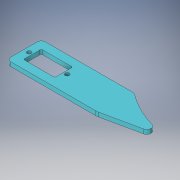
# Autodesk Inventor part: legRound
Saved by Autodesk Inventor 2019.1 (Build 231200000, 200)
## iProperties
Created: 2018-11-13
Part Number: legRound
Material: Generic
Document SubType Name: Modeling
Designer: kfortuna
Density: 1 g/cm^3
Appearance: Default
Author: kfortuna
Autodesk Inventor part; units mm, degrees
ref_plane "YZ Plane" through (0, 0, 0) normal (1, 0, 0) x (0, 1, 0)
ref_plane "XZ Plane" through (0, 0, 0) normal (0, 1, 0) x (-1, 0, 0)
ref_plane "XY Plane" through (0, 0, 0) normal (0, 0, 1) x (1, 0, 0)
sketch "Sketch1" plane through (0, 0, 0) normal (0, 1, 0) x (-1, 0, 0)
  line L0 (25.9896, 44.1273) -> (5.2671, 44.1273)
  line L1 (4.2671, 43.1273) -> (4.2671, 32.1273)
  line L2 (5.2671, 31.1273) -> (25.9896, 31.1273)
  line L3 (26.9896, 32.1273) -> (26.9896, 43.1273)
  line L4 (29.9896, 50.1273) -> (-31.3027, 50.1273)
  line L5 (-32.806, 25.1273) -> (29.9896, 25.1273)
  line L6 (32.9896, 28.1273) -> (32.9896, 47.1273)
  line L7 (-33.3897, 49.9071) -> (-60.206, 44.1846)
  arc A0 (-35.8175, 26.1359) -> (-60.3814, 38.2573) centre (-79.9609, -32.3705) ccw
  circle A1 centre (29.3148, 37.6273) radius 1.5
  circle A2 centre (1.7671, 37.6273) radius 1.5
  arc A3 (32.9896, 47.1273) -> (29.9896, 50.1273) centre (29.9896, 47.1273) ccw
  arc A4 (29.9896, 25.1273) -> (32.9896, 28.1273) centre (29.9896, 28.1273) ccw
  arc A5 (26.9896, 43.1273) -> (25.9896, 44.1273) centre (25.9896, 43.1273) ccw
  arc A6 (25.9896, 31.1273) -> (26.9896, 32.1273) centre (25.9896, 32.1273) ccw
  arc A7 (4.2671, 32.1273) -> (5.2671, 31.1273) centre (5.2671, 32.1273) ccw
  arc A8 (5.2671, 44.1273) -> (4.2671, 43.1273) centre (5.2671, 43.1273) ccw
  arc A9 (-35.8175, 26.1359) -> (-32.806, 25.1273) centre (-32.806, 30.1273) ccw
  arc A10 (-31.3027, 50.1273) -> (-33.3897, 49.9071) centre (-31.3027, 40.1273) ccw
  line L8 (-62.58, 41.2506) -> (-62.58, 41.1483)
  arc A11 (-60.206, 44.1846) -> (-62.58, 41.2506) centre (-59.58, 41.2506) ccw
  arc A12 (-62.58, 41.1483) -> (-60.3814, 38.2573) centre (-59.58, 41.1483) ccw
  point P0 (0, 0)
  point P1 (26.9896, 44.1273)
  point P2 (4.2671, 31.1273)
  point P3 (4.2671, 44.1273)
  point P4 (26.9896, 31.1273)
  point P5 (32.9896, 50.1273)
  point P6 (-34.5115, 25.1273)
  point P7 (-32.3578, 50.1273)
  point P8 (32.9896, 25.1273)
  point P9 (-62.58, 38.8302)
  dimension "d0" = 13
  dimension "d1" = 6
  dimension "d2" = 6
  dimension "d3" = 3
  dimension "d4" = 12.5
  dimension "d5" = 12.5
  dimension "d6" = 6
  dimension "d7" = 3
  dimension "d8" = 3
  dimension "d9" = 1
  dimension "d10" = 3
  dimension "d11" = 1
  dimension "d12" = 1
  dimension "d13" = 5
  dimension "d14" = 10
  dimension "d15" = 3
  dimension "d16" = 3
  constraints: 24 point on circle, 20 tangent, 18 end point, 16 point on line, 13 centre point, 3 parallel, 2 horizontal, 1 equal radius, 1 perpendicular, 1 vertical
  measures "d0" distance of point (26.99, 31.127) point (26.99, 44.127)
  measures "d1" distance between parallel lines of L4 L0
  measures "d2" distance between parallel lines of L5 L2
  measures "d3" diameter of A1
  measures "d4" distance from line of L4 A1.centre
  measures "d5" distance from line of L4 A2.centre
  measures "d6" distance between parallel lines of L6 L3
  measures "d7" radius of A3
  measures "d8" radius of A4
  measures "d9" radius of A5
  measures "d10" diameter of A2
  measures "d11" radius of A6
  measures "d12" radius of A7
  measures "d13" radius of A9
  measures "d14" radius of A10
  measures "d15" radius of A11
  measures "d16" radius of A12
extrude "Extrusion1" add sketch "Sketch1" along normal blind 3.0988
body "Solid1"
